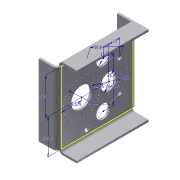
# Autodesk Inventor part: GearboxPlate
Saved by Autodesk Inventor 2013 SP1 (Build 170176100, 176)
## iProperties
Created: 2013-12-02
Part Number: GearboxPlate
Material: Aluminum 6061
Document SubType Name: Sheet Metal
Designer: robotics
Density: 2.71 g/cm^3
Sheet Metal Rule: 3mm Aluminum
Author: robotics
Autodesk Inventor part; units mm, degrees
ref_plane "YZ Plane" through (0, 0, 0) normal (1, 0, 0) x (0, 1, 0)
ref_plane "XZ Plane" through (0, 0, 0) normal (0, 1, 0) x (-1, 0, 0)
ref_plane "XY Plane" through (0, 0, 0) normal (0, 0, 1) x (1, 0, 0)
sketch "Sketch1" plane through (0, 0, 0) normal (1, 0, 0) x (0, 1, 0)
  line L0 (-45, 45) -> (45, 45)
  line L1 (45, 45) -> (45, -45)
  line L2 (45, -45) -> (-45, -45)
  line L3 (-45, -45) -> (-45, 45)
  point P0 (0, 0)
  dimension "d0" = 90
  dimension "d35" = 90
  dimension "d36" = 45
  dimension "d37" = 45
  measures "d0" distance of L0.start L0.end
  measures "d35" distance of L0.end L1.end
  measures "d36" distance from line of L1 point (0, 0)
  measures "d37" distance from line of L0 point (0, 0)
extrude "Plate1" add sketch "Sketch1" along normal blind 3
sketch "Sketch2" plane through (-3, 48, -45) normal (0, 1, 0) x (-1, 0, 0)
  line L0 (0, 90) -> (0, 0)
  line L1 (0, 0) -> (19, 0)
  line L2 (19, 0) -> (19, 90)
  line L3 (19, 90) -> (0, 90)
  constraints: 6 end point, 1 horizontal, 1 perpendicular, 1 vertical
edge flange "Flange1" height 25 angle 90 thickness 3 bend radius 3 thickness toward (0, 1, 0) relief straight relief width 3 relief depth 1.5 corner gap 3 corner form 0 edges at (0, 45, 0) (0, -45, 0) wall of the first edge with corners at (-3, 48, 45) (-3, 48, -45) (-22, 48, -45) (-22, 48, 45)
bend "Bend1"
corner "Corner1"
sketch "Sketch3" plane through (6, -45, 48) normal (0, 0, 1) x (1, 0, 0)
  line L0 (0, 90) -> (0, 0)
  line L1 (0, 0) -> (19, 0)
  line L2 (19, 0) -> (19, 90)
  line L3 (19, 90) -> (0, 90)
  constraints: 6 end point, 1 horizontal, 1 perpendicular, 1 vertical
edge flange "Flange2" height 25 angle 90 thickness 3 bend radius 3 thickness toward (0, 0, 1) relief straight relief width 3 relief depth 1.5 corner gap 3 corner form 0 edges at (3, 0, 45) (3, 0, -45) wall of the first edge with corners at (6, 45, 48) (6, -45, 48) (25, -45, 48) (25, 45, 48)
bend "Bend2"
corner "Corner2"
sketch "Sketch4" plane through (3, 0, 0) normal (1, 0, 0) x (0, 0, -1)
  line L0 (-45, 45) -> (45, 45) projected
  line L1 (-45, -45) -> (-45, 45) projected
  line L2 (45, -45) -> (-45, -45) projected
  line L3 (45, 45) -> (45, -45) projected
  circle A0 centre (-29.9989, 7.3061) radius 7.62 construction
  circle A1 centre (1.5, 17.4637) radius 12.7 construction
  circle A2 centre (32.9989, 7.3061) radius 7.62 construction
  circle A3 centre (1.5, -20.7125) radius 25.4 construction
  circle A4 centre (1.5, 17.4637) radius 25.4 construction
  line L4 (25.7467, 9.6448) -> (25.6742, 9.6682) construction
  line L5 (-22.7467, 9.6448) -> (-22.6742, 9.6682) construction
  line L6 (1.5, 4.6875) -> (1.5, 4.7637) construction
  line L7 (-33.5, -17.8514) -> (-26.4979, 32.4637) construction
  line L8 (36.5, -17.8514) -> (29.4979, 32.4637) construction
  point P0 (0, 0)
  dimension "d24" = 25.4
  dimension "d25" = 15.24
  dimension "d27" = 50.8
  dimension "d23" = 0.0762
  dimension "d26" = 50.8
  dimension "d34" = 62.9979
  dimension "d38" = 24.2875
  dimension "d40" = 46.5
  dimension "d41" = 43.5
  dimension "d42" = 50.8
  dimension "d43" = 15
  dimension "d45" = 70
  constraints: 10 end point, 3 coincident, 3 equal length, 3 vertical alignment, 2 horizontal alignment, 2 line through centre, 2 midpoint, 2 point on circle, 2 vertical, 1 centre point, 12 other
  measures "d23" distance of L6.start L6.end
  measures "d26" diameter of A4
  measures "d34" distance of point (32.999, 7.306) point (-29.999, 7.306)
  measures "d38" distance from line of L2 point (1.5, -20.712)
  measures "d40" distance from line of L1 point (1.5, 17.464)
  measures "d41" distance from line of L3 point (1.5, 17.464)
  measures "d42" distance of L7.start L7.end
  measures "d43" vertical distance of point (1.5, 17.464) L7.end
  measures "d45" distance of L8.start L7.start
sketch "Sketch5" plane through (3, 0, 0) normal (1, 0, 0) x (0, 0, -1)
  circle A0 centre (-29.9989, 7.3061) radius 9.525
  circle A1 centre (32.9989, 7.3061) radius 9.525
  circle A2 centre (1.5, 17.4637) radius 11.1125
  circle A3 centre (1.5, -20.7125) radius 14.2875
  line L0 (-33.5, -17.8514) -> (-26.4979, 32.4637) construction
  line L1 (36.5, -17.8514) -> (29.4979, 32.4637) construction
  circle A4 centre (-26.4979, 32.4637) radius 3
  circle A5 centre (29.4979, 32.4637) radius 3
  circle A6 centre (36.5, -17.8514) radius 3
  circle A7 centre (-33.5, -17.8514) radius 3
  point P0 (0, 0)
  dimension "d28" = 19.05
  dimension "d30" = 22.225
  dimension "d31" = 28.575
  dimension "d44" = 6
  constraints: 8 centre point, 8 coincident, 4 equal radius
  measures "d28" diameter of A0
  measures "d30" diameter of A2
  measures "d31" diameter of A3
  measures "d44" diameter of A5
extrude "Cut1" cut sketch "Sketch5" against normal blind 3
equation "\"d32\" = Thickness"
equation "\"d3\" = BendReliefWidth"
equation "\"d4\" = BendReliefDepth"
equation "\"d5\" = MinimumRemnant"
equation "\"d6\" = BendRadius"
equation "\"d9\" = BendRadius"
equation "\"d10\" = CornerReliefSize"
equation "\"d11\" = GapSize"
equation "\"d12\" = JacobiRadiusSize"
equation "\"d13\" = BendReliefWidth"
equation "\"d14\" = BendReliefDepth"
equation "\"d15\" = MinimumRemnant"
equation "\"d16\" = BendRadius"
equation "\"d19\" = BendRadius"
equation "\"d20\" = CornerReliefSize"
equation "\"d21\" = GapSize"
equation "\"d22\" = JacobiRadiusSize"
equation "\"d36\" = 0.5 * d0"
equation "\"d37\" = 0.5 * d35"
equation "\"BendRadius\" = Thickness"
equation "\"BendReliefWidth\" = Thickness"
equation "\"BendReliefDepth\" = 0.5 * Thickness"
equation "\"CornerReliefSize\" = 4 * Thickness"
equation "\"MinimumRemnant\" = 2 * Thickness"
equation "\"TransitionRadius\" = BendRadius"
equation "\"JacobiRadiusSize\" = BendRadius"
equation "\"GapSize\" = Thickness"
equation "\"d2\" = BendRadius"
equation "\"Thickness\" = 3"
body "Solid1"
